Autodesk Fusion 360 part; units mm, degrees
note: some values were not read from the file. Set by a fixed rule: which face or edge a step refers to.
(part 2 of 2)
sketch "Sketch1 (3)" plane through (-1.1245, 0, 0) normal (-1, 0, 0) x (0, -1, 0) in component "holder-v2"
  circle A0 centre (-14.3886, 35.5123) radius 3.2
  circle A1 centre (-14.3886, 35.5123) radius 7.5
  line L0 (5.6114, 28.0123) -> (-14.3886, 28.0123)
  line L1 (-14.3886, 28.0123) -> (-24.3886, 10.6918)
  line L2 (-24.3886, 10.6918) -> (-14.3886, -6.6287)
  line L3 (-14.3886, -6.6287) -> (5.6114, -6.6287)
  line L4 (5.6114, -6.6287) -> (15.6114, 10.6918)
  line L5 (15.6114, 10.6918) -> (5.6114, 28.0123)
  line L6 (-44.698, 23.3879) -> (15.9208, 23.3879)
  line L7 (-14.3886, 43.0123) -> (-14.3886, 28.0123) construction
  line L8 (-32.3886, 23.3879) -> (-32.3886, 40.7085) construction
  line L9 (-23.0488, 43.0123) -> (-41.7091, 10.6918)
  line L10 (-41.7091, 10.6918) -> (-23.0488, -21.6287)
  line L11 (-23.0488, -21.6287) -> (14.2717, -21.6287)
  line L12 (14.2717, -21.6287) -> (32.9319, 10.6918)
  line L13 (32.9319, 10.6918) -> (14.2717, 43.0123)
  line L14 (14.2717, 43.0123) -> (-23.0488, 43.0123)
  line L15 (-41.7091, 10.6918) -> (32.9319, 10.6918) construction
  circle A2 centre (-14.3886, -14.1287) radius 7.5
  line L16 (-21.8886, 75.5123) -> (-6.8886, 75.5123)
  line L17 (-49.2662, -28.7364) -> (22.1891, -28.7364)
  line L18 (-21.8886, -14.1287) -> (-21.8886, -28.7364)
  line L19 (-8.3876, 20.0379) -> (-8.3876, 5.2379)
  line L20 (-6.8886, -14.1287) -> (-6.8886, -28.7364)
  line L21 (-21.8886, -23.7364) -> (-6.8886, -23.7364)
  point P0 (-14.3886, 35.5123)
  point P1 (-4.3886, 10.6918)
  dimension "d314" = 6.4
  dimension "d315" = 15
  dimension "d316" = 20
  dimension "d317" = 15
  dimension "d320" = 52.1244
  dimension "d321" = 52.1244
  dimension "d324" = 5
  constraint coincident P0 A0.centre
  constraint concentric A0 A1
  constraint parallel L0 L6
  constraint parallel L7 L8
  constraint coincident P0 L7
  constraint coincident A1 L0.end
  constraint coincident A1 L7.start
  constraint coincident L0.end L1.start
  constraint symmetric A1 L15 A2
  constraint parallel L11 L17
  constraint parallel L18 L19
  constraint tangent A2 L18
  constraint parallel L18 L20
  constraint tangent A2 L20
  constraint coincident A2 L18.start
  constraint coincident A2 L20.start
  constraint coincident L17 L18.end
  constraint coincident L17 L20.end
  constraint coincident L18 L21.start
  constraint coincident L20 L21.end
  constraint perpendicular L20 L21
  measures "d314" diameter of A0
  measures "d315" diameter of A1
  measures "d316" distance of L0.start P1
  measures "d320" distance of L6 L16
  measures "d321" distance of L6 L17
  measures "d324" distance of L17 L21
extrude "Extrude1''''" add sketch "Sketch1 (3)" along normal blind 4 separate body contours A0 | A1 | A1 L0 L3 L4 L5 L11 L12 L13 L14 A2 L20 | A2 | L11 A2 L20 | L11 A2 L18 | L11 L18 L20 L21 | L17 L18 L20 L21 makes body 23 in component "holder-v2"
mirror "Mirror1''" about plane through (36.4957, 14.3886, 80.5123) normal (1, 0, 0) of bodies 23 makes body 24 in component "holder-v2"
extrude "Extrude2''''" add sketch "Sketch1 (3)" against normal up to surface (75.2404 mm away) contours L17 L18 L20 L21 bodies 23 24 in component "holder-v2"
sketch "Sketch2 (5)" plane through (0, 0, -28.7364) normal (0, 0, -1) x (1, 0, 0) in component "holder-v2"
  line L0 (78.1158, -6.8886) -> (-5.1245, -6.8886)
  line L1 (-5.1245, -6.8886) -> (-5.1245, -21.8886)
  line L2 (-5.1245, -21.8886) -> (78.1158, -21.8886)
  line L3 (78.1158, -21.8886) -> (78.1158, -6.8886)
  line L4 (-5.1245, -6.8886) -> (78.1158, -21.8886) construction
  circle A0 centre (36.4957, -14.3886) radius 3.2
  dimension "d327" = 6.4
  constraint coincident L0.end L1.start
  constraint coincident L2.end L3.start
  constraint midpoint L4 A0.centre
  measures "d327" diameter of A0
extrude "Extrude3''''" cut sketch "Sketch2 (5)" against normal up to surface (5 mm away) contours A0 bodies 23 in component "holder-v2"
sketch "Sketch3 (6)" plane through (78.1158, 0, 0) normal (1, 0, 0) x (0, 1, 0) in component "holder-v2"
  line L0 (21.8886, -28.7364) -> (21.8886, -14.1287)
  arc A0 (21.8886, -14.1287) -> (14.3886, -6.6287) centre (14.3886, -14.1287) ccw
  line L1 (14.3886, -6.6287) -> (-5.6114, -6.6287)
  line L2 (-5.6114, -6.6287) -> (-15.6114, 10.6918)
  line L3 (-15.6114, 10.6918) -> (-5.6114, 28.0123)
  line L4 (-5.6114, 28.0123) -> (14.3886, 28.0123)
  arc A1 (14.3886, 28.0123) -> (14.3886, 43.0123) centre (14.3886, 35.5123) ccw
  line L5 (14.3886, 43.0123) -> (-14.2717, 43.0123)
  line L6 (-14.2717, 43.0123) -> (-32.9319, 10.6918)
  line L7 (-32.9319, 10.6918) -> (-14.2717, -21.6287)
  line L8 (-14.2717, -21.6287) -> (6.8886, -21.6287)
  line L9 (6.8886, -21.6287) -> (6.8886, -28.7364)
  line L10 (6.8886, -28.7364) -> (21.8886, -28.7364)
  circle A2 centre (14.3886, 35.5123) radius 3.2
  dimension "d335" = 6.4
  constraint concentric A1 A2
  measures "d335" diameter of A2
sketch "Sketch4 (4)" plane through (0, 0, 75.5123) normal (0, 0, 1) x (-1, 0, 0) in component "panel"
  circle A0 centre (-36.4957, -14.3886) radius 3.15
  line L0 (-78.1158, -21.8886) -> (5.1245, -21.8886)
  line L1 (5.1245, -21.8886) -> (5.1245, -6.8886)
  line L2 (5.1245, -6.8886) -> (-78.1158, -6.8886)
  line L3 (-78.1158, -6.8886) -> (-78.1158, -21.8886)
  line L4 (-49.9957, -37.7713) -> (-22.9957, -37.7713)
  line L5 (-22.9957, -37.7713) -> (-9.4957, -14.3886)
  line L6 (-9.4957, -14.3886) -> (-22.9957, 8.9941)
  line L7 (-22.9957, 8.9941) -> (-49.9957, 8.9941)
  line L8 (-49.9957, 8.9941) -> (-63.4957, -14.3886)
  line L9 (-63.4957, -14.3886) -> (-49.9957, -37.7713)
  point P0 (-36.4957, -14.3886)
  dimension "d291" = 27
  constraint coincident P0 A0.centre
  constraint parallel L2 L7
  measures "d291" distance of L4.start P0
extrude "Extrude7''''" add sketch "Sketch4 (4)" along normal blind 10 separate body contours A0 | L0 L2 L5 L6 L8 L9 | L0 L4 L5 L9 | L2 L6 L7 L8 makes body 25 in component "panel"
sketch "Sketch5 (3)" plane through (0, 0, 85.5123) normal (0, 0, 1) x (-1, 0, 0) in component "panel"
  line L0 (-63.4957, -14.3886) -> (-49.9957, -37.7713)
  line L1 (-49.9957, -37.7713) -> (-22.9957, -37.7713)
  line L2 (-22.9957, -37.7713) -> (-9.4957, -14.3886)
  line L3 (-9.4957, -14.3886) -> (-22.9957, 8.9941)
  line L4 (-22.9957, 8.9941) -> (-49.9957, 8.9941)
  line L5 (-49.9957, 8.9941) -> (-63.4957, -14.3886)
  line L6 (-41.4753, -17.2636) -> (-36.4957, -20.1386)
  line L7 (-36.4957, -20.1386) -> (-31.516, -17.2636)
  line L8 (-31.516, -17.2636) -> (-31.516, -11.5136)
  line L9 (-31.516, -11.5136) -> (-36.4957, -8.6386)
  line L10 (-36.4957, -8.6386) -> (-41.4753, -11.5136)
  line L11 (-41.4753, -11.5136) -> (-41.4753, -17.2636)
  line L12 (-78.1158, -6.8886) -> (-78.1158, -21.8886)
  circle A0 centre (-36.4957, -14.3886) radius 3.15
  point P0 (-36.4957, -14.3886)
  point P1 (-36.4957, -14.3886)
  dimension "d294" = 5.75
  dimension "d295" = 6.3
  constraint coincident P1 P0
  constraint parallel L11 L12
  measures "d294" distance of L6.start P1
  measures "d295" diameter of A0
extrude "Extrude8''" cut sketch "Sketch5 (3)" against normal up to surface (10 mm away) contours A0 bodies 25 in component "panel"
extrude "Extrude9'" cut sketch "Sketch5 (3)" against normal blind 6 contours L6 L7 L8 L9 L10 L11 bodies 25 in component "panel"
sketch "Sketch6 (4)" plane through (0, 0, 75.5123) normal (0, 0, -1) x (1, 0, 0) in component "panel"
  circle A0 centre (36.4957, -14.3886) radius 3.15
  line L0 (49.9957, -37.7713) -> (63.4957, -14.3886)
  line L1 (63.4957, -14.3886) -> (49.9957, 8.9941)
  line L2 (49.9957, 8.9941) -> (22.9957, 8.9941)
  line L3 (22.9957, 8.9941) -> (9.4957, -14.3886)
  line L4 (9.4957, -14.3886) -> (22.9957, -37.7713)
  line L5 (22.9957, -37.7713) -> (49.9957, -37.7713)
  line L6 (22.9957, 8.9941) -> (36.4957, -14.3886) construction
  circle A1 centre (27.7506, 0.7584) radius 2
  circle A2 centre (27.7506, 0.7584) radius 5.2
  circle A3 centre (19.0055, -14.3886) radius 2
  circle A4 centre (19.0055, -14.3886) radius 5.2
  circle A5 centre (27.7506, -29.5355) radius 2
  circle A6 centre (27.7506, -29.5355) radius 5.2
  circle A7 centre (45.2407, -29.5355) radius 2
  circle A8 centre (45.2407, -29.5355) radius 5.2
  circle A9 centre (53.9858, -14.3886) radius 2
  circle A10 centre (53.9858, -14.3886) radius 5.2
  circle A11 centre (45.2407, 0.7584) radius 2
  circle A12 centre (45.2407, 0.7584) radius 5.2
  dimension "d300" = 4
  dimension "d301" = 10.4
  dimension "d303" = 360
  constraint coincident L2.end L3.start
  constraint coincident A0.centre L6.end
  constraint concentric A1 A2
  constraint coincident L6 A1.centre
  measures "d300" diameter of A1
  measures "d301" diameter of A2
extrude "Extrude10'" cut sketch "Sketch6 (4)" against normal up to surface (10 mm away) contours A1 | A3 | A5 | A7 | A9 | A11 bodies 25 in component "panel"
extrude "Extrude11'" cut sketch "Sketch6 (4)" against normal blind 4 contours A2 | A4 | A6 | A8 | A10 | A12 bodies 25 in component "panel"
chamfer "Chamfer2''" distance 2 distance2 3.2 6 edges at (25.8859, -0.0351, 79.5123) (17.1408, 15.1118, 79.5123) (25.8859, 30.2587, 79.5123) (43.3761, 30.2587, 79.5123) (52.1212, 15.1118, 79.5123) (43.3761, -0.0351, 79.5123) measured on face at (29.7441, -0.5974, 83.5123) measured on face at (20.999, 14.5495, 83.5123) measured on face at (29.7441, 29.6964, 83.5123) measured on face at (47.2342, 29.6964, 83.5123) measured on face at (55.9793, 14.5495, 83.5123) measured on face at (47.2342, -0.5974, 83.5123) on bodies 25 in component "panel"
fillet "Fillet3" radius 1 18 edges at (36.4957, 37.7713, 85.5123) (16.2457, 26.0799, 85.5123) (16.2457, 2.6972, 85.5123) (36.4957, -8.9941, 85.5123) (56.7457, 2.6972, 85.5123) (56.7457, 26.0799, 85.5123) (56.7457, 26.0799, 75.5123) (36.4957, 37.7713, 75.5123) (16.2457, 26.0799, 75.5123) (16.2457, 2.6972, 75.5123) (36.4957, -8.9941, 75.5123) (56.7457, 2.6972, 75.5123) (49.9957, -8.9941, 80.5123) (63.4957, 14.3886, 80.5123) (49.9957, 37.7713, 80.5123) (22.9957, -8.9941, 80.5123) (22.9957, 37.7713, 80.5123) (9.4957, 14.3886, 80.5123) on bodies 25 in component "panel"
fillet "Fillet4" radius 0.5 6 edges at (40.3926, -2.6388, 75.5123) (22.9025, -2.6388, 75.5123) (14.1574, 12.5082, 75.5123) (22.9025, 27.6551, 75.5123) (40.3926, 27.6551, 75.5123) (49.1377, 12.5082, 75.5123) on bodies 25 in component "panel"
sketch "Sketch4 (5)" plane through (74.1158, 0, 0) normal (-1, 0, 0) x (0, -1, 0) in component "holder-v2"
  line L0 (-21.8886, -23.7364) -> (-6.8886, -23.7364)
  line L1 (-6.8886, -23.7364) -> (-6.8886, -21.6287)
  line L2 (-6.8886, -21.6287) -> (14.2717, -21.6287)
  line L3 (14.2717, -21.6287) -> (32.9319, 10.6918)
  line L4 (32.9319, 10.6918) -> (14.2717, 43.0123)
  line L5 (14.2717, 43.0123) -> (-14.3886, 43.0123)
  arc A0 (-14.3886, 43.0123) -> (-14.3886, 28.0123) centre (-14.3886, 35.5123) ccw
  line L6 (-14.3886, 28.0123) -> (5.6114, 28.0123)
  line L7 (5.6114, 28.0123) -> (15.6114, 10.6918)
  line L8 (15.6114, 10.6918) -> (5.6114, -6.6287)
  line L9 (5.6114, -6.6287) -> (-14.3886, -6.6287)
  arc A1 (-14.3886, -6.6287) -> (-21.8886, -14.1287) centre (-14.3886, -14.1287) ccw
  line L10 (-21.8886, -14.1287) -> (-21.8886, -23.7364)
  circle A2 centre (-14.3886, 35.5123) radius 3.2
  dimension "d338" = 6.4
  constraint concentric A0 A2
  measures "d338" diameter of A2
extrude "Extrude7'''''" add sketch "Sketch4 (5)" along normal blind 2 contours A2 bodies 23 in component "holder-v2"
extrude "Extrude8'''" add 1 faces at (72.1158, 14.7902, 36.3463) along direction (-1, 0, 0) blind 3.2 on bodies 23 bodies 23 in component "holder-v2"
chamfer "Chamfer2'''" distance 3.2 angle 45 1 edges at (68.9158, 17.372, 34.3551) on bodies 23 in component "holder-v2"
extrude "Extrude9''" cut sketch "Sketch1 (3)" along normal up to surface (4 mm away) contours A0 bodies 23 in component "holder-v2"
fillet "Fillet2'" radius 1 22 edges at (78.1158, 21.8886, 55.5123) (78.1158, 14.3886, 28.0123) (78.1158, 6.8886, 55.5123) (-5.1245, 21.8886, 55.5123) (-5.1245, 14.3886, 28.0123) (-5.1245, 6.8886, 55.5123) (-1.1245, 6.8886, 49.5123) (-1.1245, 14.3886, 28.0123) (-1.1245, 21.8886, 49.5123) (74.1158, 21.8886, 49.5123) (74.1158, 14.3886, 28.0123) (74.1158, 6.8886, 49.5123) (78.1158, 14.3886, 75.5123) (36.4957, 6.8886, 75.5123) (36.4957, 21.8886, 75.5123) (-5.1245, 14.3886, 75.5123) (36.4957, 21.8886, 70.5123) (70.6158, 21.8886, 67.0123) (70.6158, 6.8886, 67.0123) (36.4957, 6.8886, 70.5123) (2.3755, 6.8886, 67.0123) (2.3755, 21.8886, 67.0123) on bodies 20 in component "holder"
fillet "Fillet1''" radius 1 54 edges at (-3.1245, 6.8886, -21.6287) (76.1158, 6.8886, -21.6287) (78.1158, -3.6916, -21.6287) (-5.1245, -3.6916, -21.6287) (-1.1245, -3.6916, -21.6287) (74.1158, -3.6916, -21.6287) (76.1158, -14.2717, -21.6287) (-3.1245, -14.2717, -21.6287) (78.1158, 4.3886, -6.6287) (78.1158, 19.6919, -8.8254) (78.1158, 21.8886, -21.4326) (78.1158, -10.6114, 2.0315) (78.1158, -10.6114, 19.352) (78.1158, 0.0584, 43.0123) (78.1158, 21.8886, 35.5123) (78.1158, 4.3886, 28.0123) (74.1158, 4.3886, 28.0123) (74.1158, 21.8886, 35.5123) (74.1158, 0.0584, 43.0123) (78.1158, -23.6018, 26.852) (74.1158, -23.6018, 26.852) (78.1158, -23.6018, -5.4685) (74.1158, -23.6018, -5.4685) (76.1158, -32.9319, 10.6918) (76.1158, -14.2717, 43.0123) (74.1158, 21.8886, -18.9326) (74.1158, 19.6919, -8.8254) (74.1158, 4.3886, -6.6287) (74.1158, -10.6114, 2.0315) (74.1158, -10.6114, 19.352) (36.4957, 6.8886, -23.7364) (36.4957, 21.8886, -23.7364) (-5.1245, 4.3886, -6.6287) (-5.1245, 19.6919, -8.8254) (-5.1245, 21.8886, -21.4326) (-1.1245, 4.3886, -6.6287) (-1.1245, 19.6919, -8.8254) (-1.1245, 21.8886, -18.9326) (-5.1245, -10.6114, 2.0315) (-1.1245, -10.6114, 2.0315) (-5.1245, -10.6114, 19.352) (-1.1245, -10.6114, 19.352) (-5.1245, 0.0584, 43.0123) (-5.1245, 21.8886, 35.5123) (-5.1245, 4.3886, 28.0123) (-1.1245, 4.3886, 28.0123) (-1.1245, 21.8886, 35.5123) (-1.1245, 0.0584, 43.0123) (-1.1245, -23.6018, 26.852) (-5.1245, -23.6018, 26.852) (-3.1245, -14.2717, 43.0123) (-3.1245, -32.9319, 10.6918) (-1.1245, -23.6018, -5.4685) (-5.1245, -23.6018, -5.4685) on bodies 23 in component "holder-v2"
fillet "Fillet1''" radius 1 5 edges at (36.4957, 21.8886, -28.7364) (36.4957, 6.8886, -28.7364) (-5.1245, 14.3886, -28.7364) (-5.1245, 6.8886, -25.1826) (78.1158, 6.8886, -25.1826) on bodies 23 in component "holder-v2"
fillet "Fillet1''" radius 1 2 edges at (-1.1245, 6.8886, -22.6826) (74.1158, 6.8886, -22.6826) on bodies 23 in component "holder-v2"
fillet "Fillet1''" radius 1 1 edges at (78.1158, 14.3886, -28.7364) on bodies 23 in component "holder-v2"
sketch "Sketch1 (4)" plane through (0, 0, 2) normal (0, 0, 1) x (-1, 0, 0)
  line L0 (-33, 18) -> (-33, -18)
  line L1 (-33, -18) -> (33, -18)
  line L2 (33, -18) -> (33, 18)
  line L3 (33, 18) -> (-33, 18)
  circle A0 centre (-20.1206, 9.8608) radius 1.75
  circle A1 centre (32.6724, 10.4263) radius 1.75
  dimension "d26" = 3.5
  dimension "d27" = 3.5
  dimension "d28" = 52.793
  measures "d26" diameter of A0
  measures "d27" diameter of A1
  measures "d28" horizontal distance of A0.centre A1.centre
component "sensor" placed x (1, 0, 0) y (0, 1, 0) z (0, 0, 1) at (1.8755, -0.6114, 3.6379)
component "enclosure" placed x (1, 0, 0) y (0, 1, 0) z (0, 0, 1) at (0, 0, 0)
component "holder" placed x (1, 0, 0) y (0, 1, 0) z (0, 0, 1) at (0, 0, 0)
component "panel" placed x (1, 0, 0) y (0, 1, 0) z (0, 0, 1) at (0, 0, 0)
component "holder-v2" placed x (-1, 0, 0) y (0, -1, 0) z (0, 0, 1) at (72.9913, 28.7771, 0)
hidden bodies 22
equation "box_width = 63 mm"
equation "box_depth = 39 mm"
equation "box_height = 36 mm"
equation "wall = 2 mm"
equation "d5 = box_width"
equation "d6 = box_depth"
equation "d7 = box_height"
equation "d9 = wall"
equation "d10 = 5 mm + 9 mm + ( 20.5 / 2 ) * 1 mm"
equation "sensor_size = 16.5 mm"
equation "sensor_dist = 25 mm"
equation "gap = 0.4 mm"
equation "d34 = 23 mm + gap"
equation "d36 = 7 mm + gap"
equation "d37 = 57 mm + 2 mm"
equation "d45 = gap"
equation "d46 = gap"
equation "d57 = wall + gap + 12.601 mm"
equation "d58 = 5 mm + 1.6 mm + 7 mm"
equation "d59 = 16 mm + 2 * gap"
equation "d60 = 14 mm + 2 * gap"
equation "d64 = sensor_size + 2 * gap"
equation "d65 = sensor_dist / 2"
equation "d72 = 21.3 mm + 2 * gap + 5 mm"
equation "d73 = 16 mm + 2 * gap"
equation "d74 = 14 mm + 2 * gap"
equation "d78 = 10.58 mm + 2 * gap"
equation "d79 = 2.54 mm + 2 * gap"
equation "d80 = 28 mm + 2 * gap"
equation "d82 = 20.5 mm + 2 * gap"
equation "d85 = ( 45.5 / 2 ) * 1 mm + gap"
equation "d88 = -( ( 45.5 / 2 ) * 1 mm + gap )"
equation "d91 = 17 mm + 2 * gap"
equation "d92 = 8 mm + gap + 1.6 mm"
equation "d104 = wall"
equation "d112 = wall"
equation "d113 = wall"
equation "d115 = wall"
equation "d157 = wall"
equation "d158 = wall"
equation "d162 = wall"
equation "snap_gap = 0.2 mm"
equation "d177 = snap_gap"
equation "d178 = snap_gap"
equation "d179 = -12 mm - wall - gap"
equation "d181 = -wall - gap - 3 mm"
equation "d185 = -12 mm - wall - gap"
equation "d187 = -wall - gap - 3 mm"
equation "d211 = ( 11.05 / 2 ) * 1 mm"
equation "d214 = 6 mm + 2 * snap_gap"
equation "d233 = 6 mm + 2 * snap_gap"
equation "holder_height = 40 mm"
equation "d248 = holder_height"
equation "d252 = 6 mm + 2 * snap_gap"
equation "d258 = screw_diameter"
equation "d268 = screw_diameter"
equation "d269 = screw_diameter"
equation "screw_diameter = 6.3 mm"
equation "d295 = screw_diameter"
equation "d321 = d320"
equation "d341 = ( 6.4 / 2 ) * 1 mm"
equation "d343 = ( 6.4 / 2 ) * 1 mm"
named bodies: "sensorboard", "left side", "right side", "bottom", "top", "right side (1)", "left side (1)", "holder", "panel", "panel2", "holder2"
